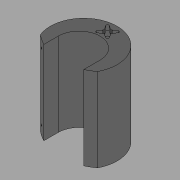
# Autodesk Inventor part: inner_mechanism
Saved by Autodesk Inventor 2019 (Build 230136000, 136)
## iProperties
Part Number: inner_mechanism
Material: Generic
Document SubType Name: Modeling
Designer: Javi
Appearance: Default
Author: Javi
Autodesk Inventor part; units mm, degrees
sketch "Sketch1" plane through (0, 0, 0) normal (0, 1, 0) x (-1, 0, 0)
  circle A0 centre (0, 0) radius 13
  arc A1 (-50, 68) -> (50, 68) centre (0, 68) ccw
  line L0 (50, 68) -> (50, 102.45)
  line L1 (-50, 68) -> (-50, 106.8831)
  arc A2 (74.4178, 86.3596) -> (50, 102.45) centre (0, 0) ccw
  circle A3 centre (0, 57) radius 80
  arc A4 (-50, 106.8831) -> (-70.6665, 94.5) centre (0, 0) ccw
  dimension "d4" = 100
  dimension "d5" = 26
  dimension "d8" = 0
  dimension "d32" = 114
  dimension "d60" = 160
  dimension "d61" = 57
  dimension "d62" = 0
  dimension "d63" = 68
  dimension "d99" = 118
  constraints: 8 point on circle, 5 centre point, 4 end point, 3 coincident, 2 tangent, 1 parallel, 1 vertical
  measures "d4" diameter of A1
  measures "d5" diameter of A0
  measures "d8" horizontal distance of A1.centre point (0, 0)
  measures "d32" radius of A2
  measures "d60" diameter of A3
  measures "d61" distance of point (0, 0) A3.centre
  measures "d62" horizontal distance of point (0, 0) A3.centre
  measures "d63" distance of point (0, 0) A1.centre
  measures "d99" radius of A4
extrude "Extrusion1" add sketch "Sketch1" along normal blind 200 contours A0 | A1 L0 A2 A3 A4 L1 picked at (-26.4774, 5.8917)
sketch "Sketch2" plane through (0, 0, 0) normal (0, -1, 0) x (1, 0, 0)
  circle A0 centre (0, 0) radius 13
  circle A1 centre (0, 0) radius 11.5
  dimension "d12" = 26
  dimension "d13" = 23
  constraints: 2 centre point, 2 coincident
  measures "d12" diameter of A0
  measures "d13" diameter of A1
extrude "Extrusion2" cut sketch "Sketch2" against normal blind 17 contours A1
sketch "Sketch3" plane through (0, 17, 0) normal (0, -1, 0) x (1, 0, 0)
  circle A0 centre (0, 0) radius 7.5
  point P0 (0, 0)
  dimension "d16" = 15
  constraints: 1 centre point, 1 coincident
  measures "d16" diameter of A0
extrude "Extrusion3" cut sketch "Sketch3" against normal blind 8
sketch "Sketch4" plane through (0, 25, 0) normal (0, -1, 0) x (1, 0, 0)
  circle A0 centre (0, 0) radius 4.5
  point P0 (0, 0)
  dimension "d19" = 9
  constraints: 1 centre point, 1 coincident
  measures "d19" diameter of A0
extrude "Extrusion4" cut sketch "Sketch4" against normal blind 163
derived "Parallax-Servo-Horn.ipt"
sketch "Sketch1_1" plane through (0, 17.3761, 0) normal (0, 0, 1) x (1, 0, 0)
  line L0 (17.8043, -15.3923) -> (7.873, -13.2486)
  line L1 (7.873, -13.2486) -> (6.3161, -13.2486)
  arc A0 (4.1275, -11.06) -> (6.3161, -13.2486) centre (6.3161, -11.06) ccw
  line L2 (4.1275, -11.06) -> (4.1275, -9.5031)
  line L3 (4.1275, -9.5031) -> (1.9838, 0.4282)
  arc A1 (1.9838, 0.4282) -> (-1.9838, 0.4282) centre (0, 0) ccw
  line L4 (-1.9838, 0.4282) -> (-4.1275, -9.5031)
  line L5 (-4.1275, -9.5031) -> (-4.1275, -11.06)
  arc A2 (-6.3161, -13.2486) -> (-4.1275, -11.06) centre (-6.3161, -11.06) ccw
  line L6 (-6.3161, -13.2486) -> (-7.873, -13.2486)
  line L7 (-7.873, -13.2486) -> (-17.8043, -15.3923)
  arc A3 (-17.8043, -15.3923) -> (-17.8043, -19.3599) centre (-17.3761, -17.3761) ccw
  line L8 (-17.8043, -19.3599) -> (-7.873, -21.5036)
  line L9 (-7.873, -21.5036) -> (-6.3161, -21.5036)
  arc A4 (-4.1275, -23.6922) -> (-6.3161, -21.5036) centre (-6.3161, -23.6922) ccw
  line L10 (-4.1275, -23.6922) -> (-4.1275, -25.2491)
  line L11 (-4.1275, -25.2491) -> (-1.9838, -35.1804)
  arc A5 (-1.9838, -35.1804) -> (1.9838, -35.1804) centre (0, -34.7522) ccw
  line L12 (1.9838, -35.1804) -> (4.1275, -25.2491)
  line L13 (4.1275, -25.2491) -> (4.1275, -23.6922)
  arc A6 (6.3161, -21.5036) -> (4.1275, -23.6922) centre (6.3161, -23.6922) ccw
  line L14 (6.3161, -21.5036) -> (7.873, -21.5036)
  line L15 (7.873, -21.5036) -> (17.8043, -19.3599)
  arc A7 (17.8043, -19.3599) -> (17.8043, -15.3923) centre (17.3761, -17.3761) ccw
  circle A8 centre (0, -9.2735) radius 0.635
  circle A9 centre (-0.0143, -6.3525) radius 0.635
  circle A10 centre (-0.0286, -3.4316) radius 0.635
  circle A11 centre (-0.0428, -0.5106) radius 0.635
  circle A12 centre (-16.8655, -17.4189) radius 0.635
  circle A13 centre (-13.9445, -17.4047) radius 0.635
  circle A14 centre (-11.0236, -17.3904) radius 0.635
  circle A15 centre (-8.1026, -17.3761) radius 0.635
  circle A16 centre (0.0428, -34.2416) radius 0.635
  circle A17 centre (0.0286, -31.3206) radius 0.635
  circle A18 centre (0.0143, -28.3997) radius 0.635
  circle A19 centre (0, -25.4787) radius 0.635
  circle A20 centre (16.8655, -17.3333) radius 0.635
  circle A21 centre (13.9445, -17.3475) radius 0.635
  circle A22 centre (11.0236, -17.3618) radius 0.635
  circle A23 centre (8.1026, -17.3761) radius 0.635
  circle A24 centre (0, -17.3761) radius 4.7016
ref_plane "Work Plane7" through (0, 197, 0) normal (0, 1, 0) x (1, 0, 0)
ref_plane "Work Plane1" through (0, 0, 114) normal (0, 0, 1) x (1, 0, 0)
ref_plane "Work Plane2" through (-74.4178, 0, 86.3596) normal (0.5502366, 0, -0.8350088) x (0, 1, 0)
ref_plane "Work Plane4" through (-62.727, 0, 95.191) normal (0.5502366, 0, -0.8350088) x (0, 1, 0)
ref_plane "Work Plane5" through (-74.4178, 0, 86.3596) normal (0.5502366, 0, -0.8350088) x (0, 1, 0)
ref_plane "Work Plane6" through (-62.727, 0, 95.191) normal (0.5502366, 0, -0.8350088) x (0, 1, 0)
sketch "Sketch13" plane through (-62.727, 0, 95.191) normal (0.5502366, 0, -0.8350088) x (0, 1, 0)
  circle A0 centre (20, -3.3787) radius 2
  line L0 (0, 14.6213) -> (200, 14.6213) projected
  line L1 (0, -14.6213) -> (0, 14.6213) projected
  circle A1 centre (180, -3.3787) radius 2
  point P0 (0, 0)
  dimension "d83" = 4
  dimension "d85" = 18
  dimension "d86" = 20
  dimension "d89" = 160
  constraints: 2 centre point, 1 horizontal, 2 other
  measures "d83" diameter of A0
  measures "d85" distance from line of L0 A0.centre
  measures "d86" distance from line of L1 A0.centre
  measures "d89" distance of A0.centre A1.centre
extrude "Extrusion11" cut sketch "Sketch13" along normal blind 16
sketch "Sketch14" plane through (0, 200, 0) normal (0, 1, 0) x (1, 0, 0)
  line L0 (11.1868, 13.9923) -> (2.6485, 8.4857)
  line L1 (2.6485, 8.4857) -> (1.5476, 7.3847)
  arc A0 (-1.5475, 7.3847) -> (1.5476, 7.3847) centre (0, 8.9323) ccw
  line L2 (-1.5475, 7.3847) -> (-2.6485, 8.4857)
  line L3 (-2.6485, 8.4857) -> (-11.1868, 13.9923)
  arc A1 (-11.1868, 13.9923) -> (-13.9923, 11.1868) centre (-12.2868, 12.2868) ccw
  line L4 (-13.9923, 11.1868) -> (-8.4857, 2.6485)
  line L5 (-8.4857, 2.6485) -> (-7.3847, 1.5475)
  arc A2 (-7.3847, -1.5475) -> (-7.3847, 1.5475) centre (-8.9323, 0) ccw
  line L6 (-7.3847, -1.5475) -> (-8.4857, -2.6485)
  line L7 (-8.4857, -2.6485) -> (-13.9923, -11.1868)
  arc A3 (-13.9923, -11.1868) -> (-11.1868, -13.9923) centre (-12.2868, -12.2868) ccw
  line L8 (-11.1868, -13.9923) -> (-2.6485, -8.4857)
  line L9 (-2.6485, -8.4857) -> (-1.5475, -7.3847)
  arc A4 (1.5476, -7.3847) -> (-1.5475, -7.3847) centre (0, -8.9323) ccw
  line L10 (1.5476, -7.3847) -> (2.6485, -8.4857)
  line L11 (2.6485, -8.4857) -> (11.1868, -13.9923)
  arc A5 (11.1868, -13.9923) -> (13.9923, -11.1868) centre (12.2868, -12.2868) ccw
  line L12 (13.9923, -11.1868) -> (8.4857, -2.6485)
  line L13 (8.4857, -2.6485) -> (7.3847, -1.5475)
  arc A6 (7.3847, 1.5475) -> (7.3847, -1.5475) centre (8.9323, 0) ccw
  line L14 (7.3847, 1.5475) -> (8.4857, 2.6485)
  line L15 (8.4857, 2.6485) -> (13.9923, 11.1868)
  arc A7 (13.9923, 11.1868) -> (11.1868, 13.9923) centre (12.2868, 12.2868) ccw
  arc A8 (70.6665, -94.5) -> (-74.4178, -86.3596) centre (0, -57) ccw projected
  line L16 (-10.6448, 14.8327) -> (-2.0168, 9.2682)
  line L17 (-2.0168, 9.2682) -> (-0.8404, 8.0918)
  arc A9 (-0.8404, 8.0918) -> (0.8404, 8.0918) centre (0, 8.9323) ccw
  line L18 (0.8404, 8.0918) -> (2.0168, 9.2682)
  line L19 (2.0168, 9.2682) -> (10.6448, 14.8327)
  arc A10 (14.8327, 10.6448) -> (10.6448, 14.8327) centre (12.2868, 12.2868) ccw
  line L20 (14.8327, 10.6448) -> (9.2682, 2.0168)
  line L21 (9.2682, 2.0168) -> (8.0918, 0.8404)
  arc A11 (8.0918, 0.8404) -> (8.0918, -0.8404) centre (8.9323, 0) ccw
  line L22 (8.0918, -0.8404) -> (9.2682, -2.0168)
  line L23 (9.2682, -2.0168) -> (14.8327, -10.6448)
  arc A12 (10.6448, -14.8327) -> (14.8327, -10.6448) centre (12.2868, -12.2868) ccw
  line L24 (10.6448, -14.8327) -> (2.0168, -9.2682)
  line L25 (2.0168, -9.2682) -> (0.8404, -8.0918)
  arc A13 (0.8404, -8.0918) -> (-0.8404, -8.0918) centre (0, -8.9323) ccw
  line L26 (-0.8404, -8.0918) -> (-2.0168, -9.2682)
  line L27 (-2.0168, -9.2682) -> (-10.6448, -14.8327)
  arc A14 (-14.8327, -10.6448) -> (-10.6448, -14.8327) centre (-12.2868, -12.2868) ccw
  line L28 (-14.8327, -10.6448) -> (-9.2682, -2.0168)
  line L29 (-9.2682, -2.0168) -> (-8.0918, -0.8404)
  arc A15 (-8.0918, -0.8404) -> (-8.0918, 0.8404) centre (-8.9323, 0) ccw
  line L30 (-8.0918, 0.8404) -> (-9.2682, 2.0168)
  line L31 (-9.2682, 2.0168) -> (-14.8327, 10.6448)
  arc A16 (-10.6448, 14.8327) -> (-14.8327, 10.6448) centre (-12.2868, 12.2868) ccw
  point P0 (0, 0)
  dimension "d4" = 100
  dimension "d5" = 26
  dimension "d8" = 0
  dimension "d32" = 114
  dimension "d60" = 160
  dimension "d61" = 57
  dimension "d62" = 0
  dimension "d63" = 68
  dimension "d99" = 118
  dimension "d102" = 2.1886
  dimension "d103" = 57
  dimension "d104" = 2.0295
  dimension "d105" = 114.361
  dimension "d106" = 90
  dimension "d107" = 8.9323
  dimension "d108" = 8.9323
  dimension "d109" = 8.9323
  dimension "d110" = 8.9323
  dimension "d111" = 11.3915
  dimension "d112" = 2.4727
  dimension "d113" = 123.4127
  dimension "d114" = 1
  constraints: 64 end point, 32 point on circle, 20 tangent, 16 centre point, 13 equal length, 12 parallel, 5 equal radius, 4 perpendicular, 23 other
  measures "d102" radius of A2
  measures "d103" distance of A8.centre point (0, 0)
  measures "d104" radius of A1
  measures "d105" angle of L4 L7
  measures "d106" angle of L6 L5
  measures "d107" distance of A2.centre point (0, 0)
  measures "d108" distance of point (0, 0) A0.centre
  measures "d109" distance of A6.centre point (0, 0)
  measures "d110" distance of A4.centre point (0, 0)
  measures "d111" distance between parallel lines of L4 L12
  measures "d112" distance from line of A8.start L12
  measures "d113" distance from line of A8.start L0
  measures "d114" distance between parallel lines of L3 L16
extrude "Extrusion12" cut sketch "Sketch14" against normal blind 12 contours A7 L15 L14 A6 L13 L12 A5 L11 L10 A4 L9 L8 A3 L7 L6 A2 L5 L4 A1 L3 L2 A0 L1 L0 | L16 L17 A9 L18 L19 A10 L20 L21 A11 L22 L23 A12 L24 L25 A13 L26 L27 A14 L28 L29 A15 L30 L31 A16
body "Solid1"
